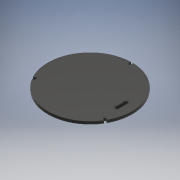
# Autodesk Inventor part: joint_lid
Saved by Autodesk Inventor 2017 (Build 210142000, 142)
## iProperties
Created: 2017-10-03
Part Number: joint_lid
Material: Acetal Resin, Black
Document SubType Name: Modeling
Designer: Thoma
Density: 1.425 g/cm^3
Appearance: Smooth - Black
Author: Thoma
Autodesk Inventor part; units mm, degrees
ref_plane "YZ Plane" through (0, 0, 0) normal (1, 0, 0) x (0, 1, 0)
ref_plane "XZ Plane" through (0, 0, 0) normal (0, 1, 0) x (-1, 0, 0)
ref_plane "XY Plane" through (0, 0, 0) normal (0, 0, 1) x (1, 0, 0)
sketch "Sketch1" plane through (0, 0, 0) normal (0, 0, 1) x (1, 0, 0)
  circle A0 centre (0, 0) radius 32
  dimension "d0" = 64
  constraints: 1 centre point, 1 coincident
  measures "d0" diameter of A0
extrude "Extrusion1" add sketch "Sketch1" along normal blind 2
sketch "Sketch2" plane through (0, 0, 2) normal (0, 0, 1) x (1, 0, 0)
  line L0 (0, 0) -> (0, 32) construction
  circle A0 centre (0, 0) radius 32 construction
  arc A1 (-0.9, 30.658) -> (0.9, 30.658) centre (0, 30.658) ccw
  line L1 (-0.9, 30.658) -> (-0.9, 31.9873)
  line L2 (0.9, 30.658) -> (0.9, 31.9873)
  circle A2 centre (0, 0) radius 32 projected
  arc A3 (0.9, 31.9873) -> (-0.9, 31.9873) centre (0, 0) ccw
  arc A4 (-26.1006, -16.1084) -> (-27.0006, -14.5496) centre (-26.5506, -15.329) ccw
  line L3 (-26.1006, -16.1084) -> (-27.2519, -16.7731)
  line L4 (-27.0006, -14.5496) -> (-28.1519, -15.2142)
  arc A5 (-28.1519, -15.2142) -> (-27.2519, -16.7731) centre (0, 0) ccw
  arc A6 (27.0006, -14.5496) -> (26.1006, -16.1084) centre (26.5506, -15.329) ccw
  line L5 (27.0006, -14.5496) -> (28.1519, -15.2142)
  line L6 (26.1006, -16.1084) -> (27.2519, -16.7731)
  arc A7 (27.2519, -16.7731) -> (28.1519, -15.2142) centre (0, 0) ccw
  point P0 (-27.7128, -16)
  point P1 (27.7128, -16)
  dimension "d3" = 30.658
  dimension "d4" = 1.8
  dimension "d7" = 360
  constraints: 15 point on circle, 14 end point, 6 centre point, 4 coincident, 3 vertical, 2 tangent, 1 point on line, 37 other
  measures "d3" distance of L0.start point (0, 30.658)
  measures "d4" diameter of A1
extrude "Extrusion2" cut sketch "Sketch2" against normal through all contours L1 A2 L2 A1 | L4 A4 L3 A2 | A2 L6 A6 L5
sketch "Sketch3" plane through (0, 0, 2) normal (0, 0, 1) x (1, 0, 0)
  line L0 (22.9, -4.5) -> (25.1, -4.5)
  line L1 (25.1, -4.5) -> (25.1, 4.5)
  line L2 (25.1, 4.5) -> (22.9, 4.5)
  line L3 (22.9, 4.5) -> (22.9, -4.5)
  line L4 (22.9, -4.5) -> (25.1, 4.5) construction
  line L5 (25.1, -4.5) -> (22.9, 4.5) construction
  circle A0 centre (0, 0) radius 28.815 construction
  point P0 (24, 0)
  dimension "d11" = 2.2
  dimension "d12" = 9
  dimension "d21" = 57.63
  dimension "d22" = 24
  constraints: 12 end point, 2 midpoint, 2 parallel, 1 centre point, 1 coincident, 1 horizontal, 1 perpendicular
  measures "d11" distance of L2.end L1.end
  measures "d12" distance of L1.end L0.end
  measures "d21" diameter of A0
  measures "d22" distance of point (24, 0) point (0, 0)
extrude "Extrusion3" cut sketch "Sketch3" against normal through all
sketch "Sketch4" plane through (0, 0, 2) normal (0, 0, 1) x (1, 0, 0)
  line L0 (25.1, 4.5) -> (25.1, -4.5) projected
  line L1 (25.1, -4.5) -> (22.9, -4.5) projected
  line L2 (22.9, -4.5) -> (22.9, 4.5) projected
  line L3 (22.9, 4.5) -> (25.1, 4.5) projected
  line L4 (-26.1006, -16.1084) -> (-27.2519, -16.7731) projected
  arc A0 (-27.2519, -16.7731) -> (27.2519, -16.7731) centre (0, 0) ccw projected
  line L5 (27.2519, -16.7731) -> (26.1006, -16.1084) projected
  arc A1 (27.0006, -14.5496) -> (26.1006, -16.1084) centre (26.5506, -15.329) ccw projected
  line L6 (27.0006, -14.5496) -> (28.1519, -15.2142) projected
  arc A2 (28.1519, -15.2142) -> (0.9, 31.9873) centre (0, 0) ccw projected
  line L7 (0.9, 31.9873) -> (0.9, 30.658) projected
  arc A3 (-0.9, 30.658) -> (0.9, 30.658) centre (0, 30.658) ccw projected
  line L8 (-0.9, 30.658) -> (-0.9, 31.9873) projected
  arc A4 (-0.9, 31.9873) -> (-28.1519, -15.2142) centre (0, 0) ccw projected
  line L9 (-28.1519, -15.2142) -> (-27.0006, -14.5496) projected
  arc A5 (-26.1006, -16.1084) -> (-27.0006, -14.5496) centre (-26.5506, -15.329) ccw projected
  line L10 (22.9, -4.5) -> (22.9, 4.5) projected
  line L11 (22.9, 0) -> (25.1, 0) construction
  arc A6 (22.9, 3.5) -> (22.9, 2.5) centre (22.9, 3) ccw
  arc A7 (22.9, -2.5) -> (22.9, -3.5) centre (22.9, -3) ccw
  line L12 (22.9, -2.5) -> (22.9, -3.5)
  line L13 (22.9, 3.5) -> (22.9, 2.5)
  dimension "d15" = 3
  dimension "d16" = 3
  dimension "d17" = 1
  dimension "d18" = 1
  constraints: 6 end point, 4 point on circle, 2 centre point, 2 coincident, 1 midpoint, 8 other
  measures "d15" distance from line of L11 point (22.9, -3)
  measures "d16" distance from line of L11 point (22.9, 3)
  measures "d17" diameter of A6
  measures "d18" diameter of A7
extrude "Extrusion4" cut sketch "Sketch4" against normal blind 1 contours L2 A6 | A7 L2
sketch "Sketch5" plane through (0, 0, 0) normal (0, 0, -1) x (-1, 0, 0)
  line L0 (-25.1, -4.5) -> (-25.1, 4.5) projected
  line L1 (-25.1, 4.5) -> (-22.9, 4.5) projected
  line L2 (-22.9, 4.5) -> (-22.9, -4.5) projected
  line L3 (-22.9, -4.5) -> (-25.1, -4.5) projected
  line L4 (27.2519, -16.7731) -> (26.1006, -16.1084) projected
  arc A0 (27.0006, -14.5496) -> (26.1006, -16.1084) centre (26.5506, -15.329) ccw projected
  line L5 (27.0006, -14.5496) -> (28.1519, -15.2142) projected
  arc A1 (28.1519, -15.2142) -> (0.9, 31.9873) centre (0, 0) ccw projected
  line L6 (0.9, 31.9873) -> (0.9, 30.658) projected
  arc A2 (-0.9, 30.658) -> (0.9, 30.658) centre (0, 30.658) ccw projected
  line L7 (-0.9, 30.658) -> (-0.9, 31.9873) projected
  arc A3 (-0.9, 31.9873) -> (-28.1519, -15.2142) centre (0, 0) ccw projected
  line L8 (-28.1519, -15.2142) -> (-27.0006, -14.5496) projected
  arc A4 (-26.1006, -16.1084) -> (-27.0006, -14.5496) centre (-26.5506, -15.329) ccw projected
  line L9 (-26.1006, -16.1084) -> (-27.2519, -16.7731) projected
  arc A5 (-27.2519, -16.7731) -> (27.2519, -16.7731) centre (0, 0) ccw projected
  line L10 (-22.9, 4.5) -> (-25.1, 4.5)
  line L11 (-25.1, 4.5) -> (-25.1, -4.5)
  line L12 (-25.1, -4.5) -> (-22.9, -4.5)
  line L13 (-22.9, -4.5) -> (-22.9, 4.5)
  line L14 (-22.9, 4.5) -> (-25.1, -4.5) construction
  line L15 (-25.1, 4.5) -> (-22.9, -4.5) construction
  line L16 (-20.9, 6.5) -> (-27.1, 6.5)
  line L17 (-27.1, 6.5) -> (-27.1, -6.5)
  line L18 (-27.1, -6.5) -> (-20.9, -6.5)
  line L19 (-20.9, -6.5) -> (-20.9, 6.5)
  circle A6 centre (0, 0) radius 28.815 construction
  point P0 (-24, 0)
  dimension "d23" = 2
  dimension "d24" = 57.63
  constraints: 20 end point, 2 midpoint, 2 parallel, 1 centre point, 1 coincident, 1 horizontal, 1 perpendicular, 3 other
  measures "d23" distance between parallel lines of L1 L16
  measures "d24" diameter of A6
extrude "Extrusion5" add sketch "Sketch5" along normal blind 2 contours L19 L18 L17 L16
body "Solid1"
